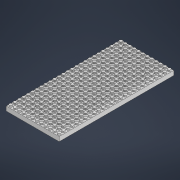
# Autodesk Inventor part: 110033226_ipt_47_船屋基地
Saved by Autodesk Inventor 2022 (Build 260153000, 153)
## iProperties
Created: 2022-06-28
Part Number: 110033226_ipt_47_船屋基地
Material: 一般
Document SubType Name: Modeling
Designer: User
Density: 1 g/cm^3
Appearance: 預設
Author: User
Autodesk Inventor part; units mm, degrees
ref_plane "YZ Plane" through (0, 0, 0) normal (1, 0, 0) x (0, 1, 0)
ref_plane "XZ Plane" through (0, 0, 0) normal (0, 1, 0) x (-1, 0, 0)
ref_plane "XY Plane" through (0, 0, 0) normal (0, 0, 1) x (1, 0, 0)
sketch "草圖1" plane through (0, 0, 0) normal (0, 1, 0) x (-1, 0, 0)
  line L0 (0, 0) -> (60, 0)
  line L1 (60, 0) -> (60, -130)
  line L2 (60, -130) -> (0, -130)
  line L3 (0, -130) -> (0, 0)
  dimension "d0" = 60
  dimension "d1" = 130
  constraints: 8 end point, 2 parallel, 1 horizontal, 1 perpendicular
  measures "d0" distance of L1.end L2.end
  measures "d1" distance of L0.end L1.end
extrude "擠出1" add sketch "草圖1" along normal blind 5
sketch "草圖2" plane through (0, 5, 0) normal (0, 1, 0) x (1, 0, 0)
  line L0 (0, 130) -> (-60, 130) projected
  line L1 (-60, 130) -> (-60, 0) projected
  line L2 (-60, 0) -> (0, 0) projected
  line L3 (0, 0) -> (0, 130) projected
  circle A0 centre (-57.5, 2.5) radius 1.7
  dimension "d4" = 3.4
  dimension "d5" = 2.5
  dimension "d6" = 2.5
  constraints: 1 centre point
  measures "d4" diameter of A0
  measures "d5" distance from line of L2 A0.centre
  measures "d6" distance from line of A0.centre L1
extrude "擠出2" add sketch "草圖2" along normal blind 1.5 contours A0
pattern_linear "矩形陣列1" count 26 spacing 5 along (0, 0, -1) count 12 spacing 5 along (1, 0, 0) of "擠出2"
